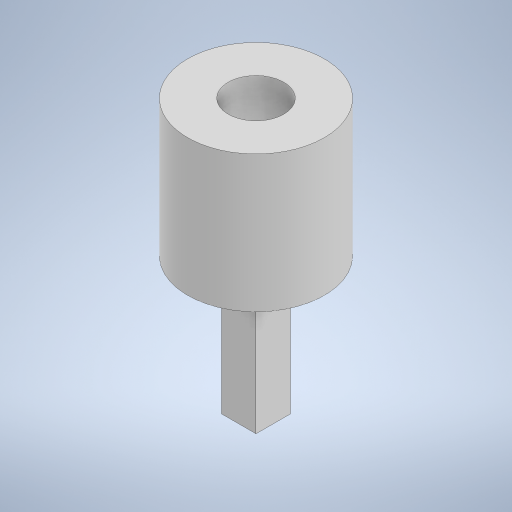
# Autodesk Inventor part: transfer
Saved by Autodesk Inventor 2024 (Build 280153000, 153)
## iProperties
Created: 2025-04-01
Part Number: transfer
Material: 一般
Document SubType Name: Modeling
Designer: TFG FabLab
Density: 1 g/cm^3
Appearance: 預設
Author: TFG FabLab
Autodesk Inventor part; units mm, degrees
ref_plane "YZ Plane" through (0, 0, 0) normal (1, 0, 0) x (0, 1, 0)
ref_plane "XZ Plane" through (0, 0, 0) normal (0, 1, 0) x (-1, 0, 0)
ref_plane "XY Plane" through (0, 0, 0) normal (0, 0, 1) x (1, 0, 0)
sketch "草圖1" plane through (0, 0, 0) normal (0, 1, 0) x (-1, 0, 0)
  circle A0 centre (0, 0) radius 7.5
  dimension "d0" = 15
  constraints: 1 centre point, 1 coincident
  measures "d0" diameter of A0
extrude "擠出1" add sketch "草圖1" along normal blind 15
sketch "草圖2" plane through (0, 15, 0) normal (0, 1, 0) x (1, 0, 0)
  circle A0 centre (0, 0) radius 3.05
  dimension "d3" = 6.1
  constraints: 1 centre point, 1 coincident
  measures "d3" diameter of A0
extrude "擠出2" cut sketch "草圖2" against normal blind 12
sketch "草圖3" plane through (0, 0, 0) normal (0, -1, 0) x (1, 0, 0)
  line L0 (1.9, 1.9) -> (-1.9, 1.9)
  line L1 (-1.9, 1.9) -> (-1.9, -1.9)
  line L2 (-1.9, -1.9) -> (1.9, -1.9)
  line L3 (1.9, -1.9) -> (1.9, 1.9)
  circle A0 centre (0, 0) radius 3.05 projected
  line L4 (1.9, 1.9) -> (-1.9, -1.9) construction
  line L5 (-1.9, 1.9) -> (1.9, -1.9) construction
  dimension "d6" = 3.8
  dimension "d7" = 3.8
  constraints: 12 end point, 2 midpoint, 2 parallel, 1 horizontal, 1 perpendicular
  measures "d6" distance of L2.end L1.end
  measures "d7" distance of L1.end L0.end
extrude "擠出3" add sketch "草圖3" along normal blind 15 contours L3 L2 L1 L0
